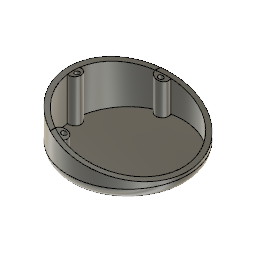
ur5_02 (Autodesk Fusion 360 archive; units mm, degrees)
design "CapUR"
part number: 2025-04-09-17-50-51-443
Autodesk Fusion 360 part; units mm, degrees
sketch "Sketch1" plane through (0, 0, 0) normal (0, 0, 1) x (1, 0, 0)
  circle A0 centre (0, 0) radius 38.1
  circle A1 centre (0, 0) radius 35.1
  dimension "d1" = 76.2
  dimension "d2" = 3
  constraint coincident A0.centre A1.centre
  constraint concentric A0 A1
  measures "d1" diameter of A0
  measures "d2" distance of A0 A1
extrude "Extrude1" add sketch "Sketch1" along normal blind 60
ref_plane "WorkPlane1" through (0, -70, 0) normal (0, 1, 0) x (0, 0, 1)
sketch "Sketch2" plane through (0, -70, 0) normal (0, 1, 0) x (1, 0, 0)
  line L0 (-38.1, -30) -> (38.1, -10)
  line L1 (-38.1, -30) -> (-38.1, -60)
  line L2 (-38.1, -60) -> (38.1, -60)
  line L3 (38.1, -60) -> (38.1, -10)
  constraint perpendicular L1 L2
  constraint perpendicular L2 L3
extrude "Extrude2" cut sketch "Sketch2" along normal blind 140
extrude "Extrude3" add sketch "Sketch1" along normal blind 2 contours A1
fillet "Fillet1" radius 8 1 edges at (-35.5217, -13.7775, 0)
sketch "Sketch3" plane through (0, 0, 2) normal (0, 0, 1) x (-1, 0, 0)
  circle A0 centre (0, 0) radius 35.1
  circle A1 centre (34, 0) radius 4
  circle A2 centre (32.55, 0) radius 1.5
  circle A3 centre (10.5066, 32.3359) radius 4
  circle A4 centre (10.0585, 30.9569) radius 1.5
  circle A5 centre (10.5066, -32.3359) radius 4
  circle A6 centre (10.0585, -30.9569) radius 1.5
  dimension "d15" = 3
  dimension "d21" = 360
  dimension "d26" = 8
  dimension "d27" = 1.45
  measures "d15" diameter of A2
  measures "d26" diameter of A1
  measures "d27" distance of A1.centre A2.centre
extrude "Extrude4" add sketch "Sketch3" along normal blind 27.19 contours A0 A1 picked at (33.932, 2.6629)
extrude "Extrude5" add sketch "Sketch3" along normal blind 22 contours A0 A3 | A0 A5 picked at (8.5086, 33.2459) picked at (8.5086, -33.2459)
sketch "Sketch4" plane through (0, -70, 0) normal (0, 1, 0) x (1, 0, 0)
  line L0 (-14.4896, -23.8029) -> (-14.4896, -24)
  line L1 (-14.4896, -24) -> (-7, -24)
  line L2 (-7, -24) -> (-6.4, -24)
  line L3 (-6.4, -24) -> (-6.4, -21.7)
  line L4 (-6.4, -21.7) -> (-14.4896, -23.8029)
  constraint vertical L0
  constraint perpendicular L0 L1
  constraint parallel L1 L2
  constraint perpendicular L1 L3
extrude "Extrude6" cut sketch "Sketch4" along normal blind 140
extrude "Extrude7" cut sketch "Sketch3" against normal blind 25 contours A2 | A4 | A6
